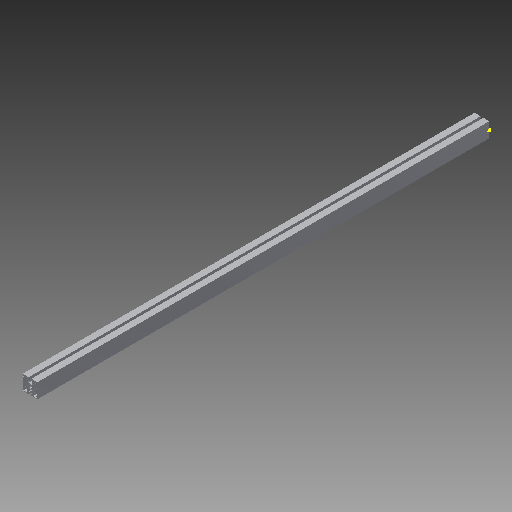
# Autodesk Inventor part: Track
Saved by Autodesk Inventor 2017 (Build 210142000, 142)
## iProperties
Created: 2012-10-08
Part Number: Track
Document SubType Name: Modeling
Designer: Administrator
Density: 2.71 g/cm^3
Material: Aluminum-6061
Description: 45X45UL 2GG
Stock Number: 20.1122 45X45UL 2GG
Appearance: Aluminum - Flat
Author: Administrator
Autodesk Inventor part; units mm, degrees
ref_plane "YZ Plane" through (0, 0, 0) normal (1, 0, 0) x (0, 1, 0)
ref_plane "XZ Plane" through (0, 0, 0) normal (0, 1, 0) x (-1, 0, 0)
ref_plane "XY Plane" through (0, 0, 0) normal (0, 0, 1) x (1, 0, 0)
sketch "Sketch1" plane through (0, 0, 0) normal (0, 0, 1) x (1, 0, 0)
  line L0 (22.5, 22.5) -> (22.5, -22.5)
  line L1 (4.1, 22.5) -> (22.5, 22.5)
  line L2 (4.1, 18) -> (4.1, 22.5)
  line L3 (6.8, 18) -> (4.1, 18)
  line L4 (6.8, 8.9213) -> (6.8, 18)
  line L5 (5.0787, 7.2) -> (6.8, 8.9213)
  line L6 (-5.0787, 7.2) -> (5.0787, 7.2)
  line L7 (-6.8, 8.9213) -> (-5.0787, 7.2)
  line L8 (-6.8, 18) -> (-6.8, 8.9213)
  line L9 (-4.1, 18) -> (-6.8, 18)
  line L10 (-22.5, -22.5) -> (-22.5, 22.5)
  line L11 (-4.1, -22.5) -> (-22.5, -22.5)
  line L12 (-4.1, -18) -> (-4.1, -22.5)
  line L13 (-6.8, -18) -> (-4.1, -18)
  line L14 (-6.8, -8.9213) -> (-6.8, -18)
  line L15 (-5.0787, -7.2) -> (-6.8, -8.9213)
  line L16 (5.0787, -7.2) -> (-5.0787, -7.2)
  line L17 (6.8, -8.9213) -> (5.0787, -7.2)
  line L18 (6.8, -18) -> (6.8, -8.9213)
  line L19 (4.1, -18) -> (6.8, -18)
  line L20 (4.1, -22.5) -> (4.1, -18)
  line L21 (22.5, -22.5) -> (4.1, -22.5)
  arc A0 (-5.2879, 3.0251) -> (-5.8, 2.813) centre (-5.5, 2.813) ccw
  line L22 (-3.7688, 1.5061) -> (-5.2879, 3.0251)
  arc A1 (-3.7688, 1.5061) -> (-3.2866, 1.5878) centre (-3.5567, 1.7183) ccw
  arc A2 (-1.5877, 3.2866) -> (-3.2866, 1.5878) centre (0, 0) ccw
  arc A3 (-1.5877, 3.2866) -> (-1.5061, 3.7688) centre (-1.7182, 3.5567) ccw
  line L23 (-3.0251, 5.2879) -> (-1.5061, 3.7688)
  arc A4 (-2.813, 5.8) -> (-3.0251, 5.2879) centre (-2.813, 5.5) ccw
  line L24 (2.813, 5.8) -> (-2.813, 5.8)
  arc A5 (3.0251, 5.2879) -> (2.813, 5.8) centre (2.813, 5.5) ccw
  line L25 (1.5061, 3.7688) -> (3.0251, 5.2879)
  arc A6 (1.5061, 3.7688) -> (1.5877, 3.2866) centre (1.7182, 3.5567) ccw
  arc A7 (3.2866, 1.5877) -> (1.5877, 3.2866) centre (0, 0) ccw
  arc A8 (3.2866, 1.5877) -> (3.7688, 1.5061) centre (3.5567, 1.7182) ccw
  line L26 (5.2879, 3.0251) -> (3.7688, 1.5061)
  arc A9 (5.8, 2.813) -> (5.2879, 3.0251) centre (5.5, 2.813) ccw
  line L27 (5.8, -2.813) -> (5.8, 2.813)
  arc A10 (5.2879, -3.0252) -> (5.8, -2.813) centre (5.5, -2.813) ccw
  line L28 (3.7688, -1.5061) -> (5.2879, -3.0252)
  arc A11 (3.7688, -1.5061) -> (3.2866, -1.5877) centre (3.5567, -1.7182) ccw
  arc A12 (1.5877, -3.2866) -> (3.2866, -1.5877) centre (0, 0) ccw
  arc A13 (1.5877, -3.2866) -> (1.5061, -3.7688) centre (1.7182, -3.5567) ccw
  line L29 (3.0251, -5.2879) -> (1.5061, -3.7688)
  arc A14 (2.813, -5.8) -> (3.0251, -5.2879) centre (2.813, -5.5) ccw
  line L30 (-2.813, -5.8) -> (2.813, -5.8)
  arc A15 (-3.0251, -5.2879) -> (-2.813, -5.8) centre (-2.813, -5.5) ccw
  line L31 (-1.5061, -3.7688) -> (-3.0251, -5.2879)
  arc A16 (-1.5061, -3.7688) -> (-1.5877, -3.2866) centre (-1.7182, -3.5567) ccw
  arc A17 (-3.2866, -1.5877) -> (-1.5877, -3.2866) centre (0, 0) ccw
  arc A18 (-3.2866, -1.5877) -> (-3.7688, -1.5061) centre (-3.5567, -1.7182) ccw
  line L32 (-5.2879, -3.0251) -> (-3.7688, -1.5061)
  arc A19 (-5.8, -2.813) -> (-5.2879, -3.0251) centre (-5.5, -2.813) ccw
  line L33 (-5.8, 2.813) -> (-5.8, -2.813)
  arc A20 (-7.2, 6.2958) -> (-7.6393, 7.3565) centre (-8.7, 6.2958) ccw
  line L34 (-7.2, -6.2958) -> (-7.2, 6.2958)
  arc A21 (-7.6393, -7.3565) -> (-7.2, -6.2958) centre (-8.7, -6.2958) ccw
  line L35 (-7.7607, -7.4778) -> (-7.6393, -7.3565)
  arc A22 (-7.7607, -7.4778) -> (-8.2, -8.5385) centre (-6.7, -8.5385) ccw
  line L36 (-8.2, -13.9151) -> (-8.2, -8.5385)
  arc A23 (-8.2, -13.9151) -> (-8.2, -15.3848) centre (-8.05, -14.65) ccw
  line L37 (-8.2, -20.1) -> (-8.2, -15.3848)
  arc A24 (-9.2, -21.1) -> (-8.2, -20.1) centre (-9.2, -20.1) ccw
  line L38 (-13.9152, -21.1) -> (-9.2, -21.1)
  arc A25 (-13.9152, -21.1) -> (-15.3849, -21.1) centre (-14.65, -21.25) ccw
  line L39 (-20.1, -21.1) -> (-15.3849, -21.1)
  arc A26 (-21.1, -20.1) -> (-20.1, -21.1) centre (-20.1, -20.1) ccw
  line L40 (-21.1, -15.3848) -> (-21.1, -20.1)
  arc A27 (-21.1, -15.3848) -> (-21.1, -13.9151) centre (-21.25, -14.65) ccw
  line L41 (-21.1, 13.9152) -> (-21.1, -13.9151)
  arc A28 (-21.1, 13.9152) -> (-21.1, 15.3849) centre (-21.25, 14.65) ccw
  line L42 (-21.1, 20.1) -> (-21.1, 15.3849)
  arc A29 (-20.1, 21.1) -> (-21.1, 20.1) centre (-20.1, 20.1) ccw
  line L43 (-15.3848, 21.1) -> (-20.1, 21.1)
  arc A30 (-15.3848, 21.1) -> (-13.9151, 21.1) centre (-14.65, 21.25) ccw
  line L44 (-9.2, 21.1) -> (-13.9151, 21.1)
  arc A31 (-8.2, 20.1) -> (-9.2, 21.1) centre (-9.2, 20.1) ccw
  line L45 (-8.2, 15.3849) -> (-8.2, 20.1)
  arc A32 (-8.2, 15.3849) -> (-8.2, 13.9152) centre (-8.05, 14.65) ccw
  line L46 (-8.2, 8.5385) -> (-8.2, 13.9152)
  arc A33 (-8.2, 8.5385) -> (-7.7606, 7.4778) centre (-6.7, 8.5385) ccw
  line L47 (-7.6393, 7.3565) -> (-7.7606, 7.4778)
  arc A34 (7.2, -6.2958) -> (7.6393, -7.3565) centre (8.7, -6.2958) ccw
  line L48 (7.2, 6.2958) -> (7.2, -6.2958)
  arc A35 (7.6393, 7.3565) -> (7.2, 6.2958) centre (8.7, 6.2958) ccw
  line L49 (7.7607, 7.4778) -> (7.6393, 7.3565)
  arc A36 (7.7607, 7.4778) -> (8.2, 8.5385) centre (6.7, 8.5385) ccw
  line L50 (8.2, 13.9151) -> (8.2, 8.5385)
  arc A37 (8.2, 13.9151) -> (8.2, 15.3848) centre (8.05, 14.65) ccw
  line L51 (8.2, 20.1) -> (8.2, 15.3848)
  arc A38 (9.2, 21.1) -> (8.2, 20.1) centre (9.2, 20.1) ccw
  line L52 (13.9152, 21.1) -> (9.2, 21.1)
  arc A39 (13.9152, 21.1) -> (15.3849, 21.1) centre (14.65, 21.25) ccw
  line L53 (20.1, 21.1) -> (15.3849, 21.1)
  arc A40 (21.1, 20.1) -> (20.1, 21.1) centre (20.1, 20.1) ccw
  line L54 (21.1, 15.3848) -> (21.1, 20.1)
  arc A41 (21.1, 15.3848) -> (21.1, 13.9151) centre (21.25, 14.65) ccw
  line L55 (21.1, -13.9152) -> (21.1, 13.9151)
  arc A42 (21.1, -13.9152) -> (21.1, -15.3849) centre (21.25, -14.65) ccw
  line L56 (21.1, -20.1) -> (21.1, -15.3849)
  arc A43 (20.1, -21.1) -> (21.1, -20.1) centre (20.1, -20.1) ccw
  line L57 (15.3848, -21.1) -> (20.1, -21.1)
  arc A44 (15.3848, -21.1) -> (13.9151, -21.1) centre (14.65, -21.25) ccw
  line L58 (9.2, -21.1) -> (13.9151, -21.1)
  arc A45 (8.2, -20.1) -> (9.2, -21.1) centre (9.2, -20.1) ccw
  line L59 (8.2, -15.3849) -> (8.2, -20.1)
  arc A46 (8.2, -15.3849) -> (8.2, -13.9152) centre (8.05, -14.65) ccw
  line L60 (8.2, -8.5385) -> (8.2, -13.9152)
  arc A47 (8.2, -8.5385) -> (7.7606, -7.4778) centre (6.7, -8.5385) ccw
  line L61 (7.6393, -7.3565) -> (7.7606, -7.4778)
  line L62 (-22.5, 22.5) -> (-4.1, 22.5)
  line L63 (-4.1, 18) -> (-4.1, 22.5)
  point P0 (-11.1716, -10.5525)
  constraints: 128 end point, 96 point on circle, 48 centre point, 2 perpendicular
extrude "Extrusion2" add sketch "Sketch1" along normal blind 1380
sketch "Sketch3" plane through (22.5, -22.5, 0) normal (1, -0.000001, 0) x (0, 0, -1)
  point P0 (0, 22.5)
body "Solid1"
